Bathroom Cabinet Foot (Autodesk Fusion 360 design; units mm, degrees)
Autodesk Fusion 360 part; units mm, degrees
note: some values were not read from the file. Set by a fixed rule: which sketch regions a step uses.
sketch "Sketch1" plane through (0, 0, 0) normal (0, 0, 1) x (1, 0, 0)
sketch "Sketch2" plane through (0, 0, 0) normal (0, 0, 1) x (1, 0, 0)
  line L0 (0, 0) -> (33, 0)
  line L1 (33, 0) -> (33, 33)
  line L2 (33, 33) -> (0, 33)
  line L3 (0, 33) -> (0, 0)
  arc A0 (33, 0) -> (0, 33) centre (-20.6429, -20.6429) ccw
  dimension "d1" = 33
  dimension "d2" = 33
  constraint horizontal L0
  constraint vertical L1
  constraint horizontal L2
  constraint vertical L3
  constraint coincident L0.start L3.end
  measures "d1" distance of L0.start L0.end
  measures "d2" distance of L0.start L2.end
extrude "Extrude1" add sketch "Sketch2" along normal blind 4.5 contours L0 L3 A0
move_face "OffsetFaces1" offset 1 3 faces at (11, 0, 1.5) (0, 22, 1.5) (21.8433, 18.069, 3)
extrude "Extrude2" cut sketch "Sketch2" along normal blind 3 from surface at 1.5 contours L0 L3 A0
fillet "Fillet1" radius 1 3 edges at (-1, -1, 2.25) (34.4371, -1, 2.25) (-1, 34.4371, 2.25)
chamfer "Chamfer1" distance 0.45 angle 45 3 edges at (0, 16.5, 4.5) (20, 20, 4.5) (16.5, 0, 4.5)
